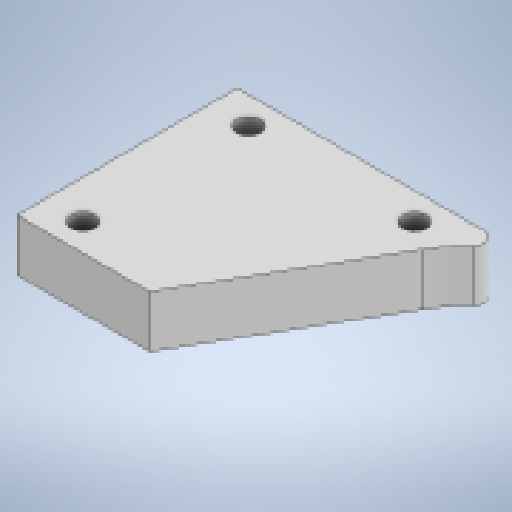
# Autodesk Inventor part: 3D_printed_part
Saved by Autodesk Inventor 2026.1 (Build 301233000, 233)
## iProperties
Created: 2025-05-14
Part Number: 3D_printed_part
Material: Generic
Document SubType Name: Modeling
Designer: User
Density: 1 g/cm^3
Appearance: Default
Author: User
Autodesk Inventor part; units mm, degrees
ref_plane "YZ Plane" through (0, 0, 0) normal (1, 0, 0) x (0, 1, 0)
ref_plane "XZ Plane" through (0, 0, 0) normal (0, 1, 0) x (-1, 0, 0)
ref_plane "XY Plane" through (0, 0, 0) normal (0, 0, 1) x (1, 0, 0)
sketch "Sketch1" plane through (0, 0, 0) normal (0, 1, 0) x (-1, 0, 0)
  line L0 (4, 10) -> (-19.4211, 10)
  line L1 (-19.4211, -10) -> (4, -10)
  line L2 (4, -10) -> (4, 10)
  arc A0 (-19.4211, -10) -> (-19.4211, 10) centre (-25.1, 0) ccw
  line L3 (4, -10) -> (6, -10)
  line L4 (6, -10) -> (6, 10)
  line L5 (6, 10) -> (4, 10)
  line L6 (4, 10) -> (4, -10)
  point P0 (0, 0)
  dimension "d0" = 20
  dimension "d2" = 4
  dimension "d3" = 10
  dimension "d6" = 10
  dimension "d7" = 23
  dimension "d8" = 29.1
  dimension "d11" = 23.4211
  dimension "d12" = 20
  dimension "d13" = 2
  constraints: 14 end point, 3 parallel, 2 horizontal, 2 point on circle, 1 centre point, 1 perpendicular
  measures "d0" distance of L1.end L0.start
  measures "d2" distance from line of point (0, 0) L2
  measures "d3" distance from line of point (0, 0) L0
  measures "d6" distance from line of L1 A0.centre
  measures "d7" diameter of A0
  measures "d8" distance from line of L2 A0.centre
  measures "d11" distance of L1.start L1.end
  measures "d12" distance of L3.end L4.end
  measures "d13" distance of L4.end L5.end
extrude "Extrusion1" add sketch "Sketch1" along normal blind 4.71
fillet "Fillet1" radius 1 2 edges at (19.4211, 2.355, -10) (19.4211, 2.355, 10)
sketch "Sketch3" plane through (0, 0, 0) normal (0, -1, 0) x (1, 0, 0)
  circle A0 centre (-2.5, -7.525) radius 1.05
  circle A1 centre (12.6, -7.525) radius 1.05
  circle A2 centre (12.6, 7.525) radius 1.05
  circle A3 centre (-2.5, 7.525) radius 1.05
  point P0 (0, 0)
  constraints: 4 centre point, 8 other
hole "Hole2" at (-2.5, 0, -7.525) at (-2.5, 0, 7.525) at (12.6, 0, 7.525) at (12.6, 0, -7.525) direction (0, 1, 0) diameter 2.1 end through all
sketch "Sketch4" plane through (0, 0, 0) normal (0, -1, 0) x (1, 0, 0)
  line L0 (1.4953, 17.8846) -> (19.0725, -12.5601)
  arc A0 (17.1193, 8.28) -> (17.1193, -8.28) centre (25.1, 0) ccw projected
  arc A1 (17.1193, 8.28) -> (16.4253, 10) centre (16.4253, 9) ccw projected
  line L1 (-6, 10) -> (16.4253, 10) projected
  point P0 (0, 0)
  point P1 (6.0474, 10)
  point P2 (15.1407, -5.75)
  dimension "d29" = 60
  constraints: 2 end point, 1 tangent
  measures "d29" angle of L1 L0
extrude "Extrusion2" cut sketch "Sketch4" against normal up to next
body "Solid1"
